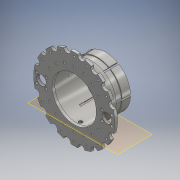
# Autodesk Inventor part: Fixture
Saved by Autodesk Inventor 2016 (Build 200138000, 138)
## iProperties
Created: 2015-07-19
Part Number: Fixture
Material: Generic
Document SubType Name: Modeling
Designer: bastli
Density: 1 g/cm^3
Appearance: Aluminum - Polished
Author: bastli
Autodesk Inventor part; units mm, degrees
ref_plane "YZ Plane" through (0, 0, 0) normal (1, 0, 0) x (0, 1, 0)
ref_plane "XZ Plane" through (0, 0, 0) normal (0, 1, 0) x (-1, 0, 0)
sketch "Sketch1" plane through (0, 0, 0) normal (0, 1, 0) x (-1, 0, 0)
  circle A0 centre (0, 0) radius 67.57
  circle A1 centre (0, 0) radius 38.25
  circle A2 centre (0, 0) radius 41.25
  circle A3 centre (0, 0) radius 36.85
  line L0 (67.57, 0) -> (-67.57, 0) construction
  line L1 (0, 67.57) -> (0, -67.57) construction
  line L2 (62.41, -8) -> (46.41, -8) construction
  line L3 (46.41, -8) -> (46.41, 8) construction
  line L4 (46.41, 8) -> (62.41, 8) construction
  line L5 (62.41, 8) -> (62.41, -8) construction
  line L6 (62.41, -8) -> (46.41, 8) construction
  line L7 (46.41, -8) -> (62.41, 8) construction
  line L8 (64.57, -10.16) -> (44.25, -10.16) construction
  line L9 (44.25, -10.16) -> (44.25, 10.16) construction
  line L10 (44.25, 10.16) -> (64.57, 10.16) construction
  line L11 (64.57, 10.16) -> (64.57, -10.16) construction
  line L12 (64.57, -10.16) -> (44.25, 10.16) construction
  line L13 (44.25, -10.16) -> (64.57, 10.16) construction
  line L14 (64.57, 0) -> (67.57, 0) construction
  line L15 (44.25, 0) -> (41.25, 0) construction
  circle A4 centre (54.41, 0) radius 7.995
  circle A5 centre (-54.41, 0) radius 7.995
  point P0 (-62.41, 8)
  point P1 (-46.41, 8)
  point P2 (-46.41, -8)
  point P3 (-62.41, -8)
  dimension "d0" = 135.14
  dimension "d1" = 76.5
  dimension "d2" = 3
  dimension "d3" = 73.7
  dimension "d4" = 16
  dimension "d5" = 16
  dimension "d6" = 20.32
  dimension "d7" = 20.32
  dimension "d30" = 15.99
  constraints: 32 end point, 9 midpoint, 8 coincident, 5 centre point, 5 symmetric about line, 4 parallel, 4 point on circle, 3 horizontal, 2 collinear, 2 perpendicular, 2 point on line, 1 horizontal alignment, 1 vertical, 3 other
  measures "d0" diameter of A0
  measures "d1" diameter of A1
  measures "d3" diameter of A3
  measures "d4" distance of L3.end L4.end
  measures "d5" distance of L4.end L2.start
  measures "d6" distance of L9.end L10.end
  measures "d7" distance of L10.end L8.start
  measures "d30" diameter of A4
extrude "Extrusion1" add sketch "Sketch1" against normal blind 4.5 contours A0 | A1 | A2 | A4 | A5
extrude "Extrusion2" add sketch "Sketch1" along normal blind 48 contours A2
ref_plane "Work Plane1" through (0, 24, 0) normal (0, 1, 0) x (1, 0, 0)
sketch "Sketch2" plane through (0, 24, 0) normal (0, 1, 0) x (1, 0, 0)
  circle A0 centre (0, 0) radius 38.25 projected
  circle A1 centre (0, 0) radius 41.25 projected
  circle A2 centre (0, 0) radius 39.75
  dimension "d14" = 1.5
  constraints: 1 centre point
  measures "d14" radial gap between concentric circles of A1 A2
extrude "Extrusion3" cut sketch "Sketch2" along normal blind 10 contours A1
sketch "Sketch3" plane through (0, 48, 0) normal (0, 1, 0) x (1, 0, 0)
  circle A0 centre (0, 0) radius 41.25 projected
  circle A1 centre (0, 0) radius 38.25 projected
  line L0 (0, 0) -> (41.25, 0) construction
  line L1 (0, 0) -> (41.2249, 1.4396) construction
  circle A2 centre (0, 0) radius 41.25 projected
  line L2 (0, 0) -> (41.2249, -1.4396) construction
  line L3 (41.2249, 1.4396) -> (38.2267, 1.3349)
  circle A3 centre (0, 0) radius 38.25 projected
  line L4 (41.2249, -1.4396) -> (38.2267, -1.3349)
  dimension "d17" = 4
  constraints: 10 end point, 7 point on circle, 2 point on line, 1 horizontal, 1 other
  measures "d17" angle of L2 L1
extrude "Extrusion4" cut sketch "Sketch3" against normal up to surface (24 mm away) contours A0 L4 A1 L3 picked at (40.2301, -1.2448)
pattern_circular "Circular Pattern1" count 6 over 360 about axis through (0, 0, 0) along (0, 1, 0) of "Extrusion4"
fillet "Fillet1" radius 3 1 edges at (41.25, 0, 0)
hole "Hole1" at (-62.41, 0, 8) at (-46.41, 0, 8) at (-46.41, 0, -8) at (-62.41, 0, -8) at (62.41, 0, 8) at (46.41, 0, 8) at (46.41, 0, -8) at (62.41, 0, -8) direction (0, -1, 0) diameter 2.4 end through all
extrude "Extrusion5" cut sketch "Sketch1" against normal through all contours A4 | A5
sketch "Sketch4" plane through (0, -4.5, 0) normal (0, -1, 0) x (1, 0, 0)
  circle A0 centre (-46.41, -8) radius 1.2 construction
  circle A1 centre (-62.41, 8) radius 1.2 construction
  circle A2 centre (-46.41, 8) radius 1.2 construction
  circle A3 centre (46.41, 8) radius 1.2 construction
  circle A4 centre (46.41, -8) radius 1.2 construction
  circle A5 centre (62.41, -8) radius 1.2 construction
  circle A6 centre (62.41, 8) radius 1.2 construction
  circle A7 centre (-62.41, -8) radius 1.2 construction
  point P0 (0, 0)
  constraints: 8 coincident
hole "Hole2" at (-62.41, -4.5, 8) at (-46.41, -4.5, 8) at (-46.41, -4.5, -8) at (-62.41, -4.5, -8) at (46.41, -4.5, -8) at (46.41, -4.5, 8) at (62.41, -4.5, 8) at (62.41, -4.5, -8) direction (0, 1, 0) diameter 4.4 depth 3 tip angle 118
sketch "Sketch5" plane through (0, 0, 0) normal (0, 1, 0) x (1, 0, 0)
  circle A0 centre (-54.41, 0) radius 7.995 construction
  circle A1 centre (54.41, 0) radius 7.995 construction
  circle A2 centre (46.41, 8) radius 1.2 construction
  circle A3 centre (62.41, -8) radius 1.2 construction
  circle A4 centre (-46.41, 8) radius 1.2 construction
  circle A5 centre (-62.41, -8) radius 1.2 construction
  circle A6 centre (-46.41, -8) radius 1.2 construction
  circle A7 centre (-62.41, 8) radius 1.2 construction
  circle A8 centre (46.41, -8) radius 1.2 construction
  circle A9 centre (62.41, 8) radius 1.2 construction
  circle A10 centre (0, 0) radius 67.57 construction
  circle A11 centre (0, 0) radius 44.25 construction
  circle A12 centre (0, 0) radius 61.57 construction
  circle A13 centre (0, 0) radius 47.25 construction
  line L0 (0, -47.25) -> (0, -61.57) construction
  line L1 (0, -47.25) -> (0, 0) construction
  circle A14 centre (54.41, 0) radius 7.995 projected
  circle A15 centre (0, 0) radius 44.25 projected
  line L2 (54.41, 0) -> (0, 0) construction
  point P0 (21.0582, -57.8569)
  point P1 (16.1605, -44.4005)
  point P2 (39.5764, -47.1654)
  point P3 (30.3717, -36.1956)
  point P4 (53.3212, -30.785)
  point P5 (40.9197, -23.625)
  point P6 (-16.1605, -44.4005)
  point P7 (-21.0582, -57.8569)
  point P8 (-30.3717, -36.1956)
  point P9 (-39.5764, -47.1654)
  point P10 (-40.9197, -23.625)
  point P11 (-53.3212, -30.785)
  point P12 (0, 61.57)
  point P13 (0, 47.25)
  point P14 (21.0582, 57.8569)
  point P15 (16.1605, 44.4005)
  point P16 (39.5764, 47.1654)
  point P17 (30.3717, 36.1956)
  point P18 (53.3212, 30.785)
  point P19 (40.9197, 23.625)
  point P20 (-16.1605, 44.4005)
  point P21 (-21.0582, 57.8569)
  point P22 (-30.3717, 36.1956)
  point P23 (-39.5764, 47.1654)
  point P24 (-40.9197, 23.625)
  point P25 (-53.3212, 30.785)
  dimension "d40" = 6
  dimension "d41" = 3
  dimension "d44" = 60
  dimension "d48" = 60
  constraints: 14 symmetric about line, 6 end point, 2 vertical, 2 vertical alignment, 1 horizontal, 18 other
hole "Hole3" at (0, 0, 61.57) at (0, 0, 47.25) at (21.0582, 0, 57.8569) at (16.1605, 0, 44.4005) at (39.5764, 0, 47.1654) at (30.3717, 0, 36.1956) at (53.3212, 0, 30.785) at (40.9197, 0, 23.625) at (-16.1605, 0, 44.4005) at (-21.0582, 0, 57.8569) at (-30.3717, 0, 36.1956) at (-39.5764, 0, 47.1654) at (-40.9197, 0, 23.625) at (-53.3212, 0, 30.785) at (40.9197, 0, -23.625) at (53.3212, 0, -30.785) at (39.5764, 0, -47.1654) at (30.3717, 0, -36.1956) at (16.1605, 0, -44.4005) at (21.0582, 0, -57.8569) at (0, 0, -47.25) at (0, 0, -61.57) at (-21.0582, 0, -57.8569) at (-16.1605, 0, -44.4005) at (-30.3717, 0, -36.1956) at (-39.5764, 0, -47.1654) at (-40.9197, 0, -23.625) at (-53.3212, 0, -30.785) direction (0, -1, 0) diameter 3.1 end through all
ref_plane "Work Plane2" through (0, 0, -41.25) normal (0, 0, 1) x (1, 0, 0)
sketch "Sketch6" plane through (0, 0, -41.25) normal (0, 0, 1) x (1, 0, 0)
  line L0 (0, 0) -> (0, 6) construction
  dimension "d57" = 6
  constraints: 2 end point, 1 vertical
  measures "d57" distance of L0.start L0.end
hole "Hole4" at (0, 6, -41.25) direction (0, 0, 1) diameter 6 end through all
sketch "Sketch7" plane through (0, 0, 0) normal (0, 1, 0) x (1, 0, 0)
  circle A0 centre (0, 0) radius 67.57 projected
  circle A1 centre (11.7334, -66.5435) radius 6
  line L0 (0, 0) -> (0, -67.57) construction
  line L1 (11.7334, -66.5435) -> (0, 0) construction
  dimension "d65" = 12
  dimension "d66" = 10
  constraints: 4 end point, 2 point on circle, 1 centre point, 1 vertical
  measures "d65" diameter of A1
  measures "d66" angle of L0 L1
extrude "Extrusion6" cut sketch "Sketch7" against normal up to surface (4.5 mm away) contours A1 A0 | A0 A1 picked at (11.6158, -64.5273) picked at (12.0898, -68.4914)
pattern_circular "Circular Pattern2" count 4 over 60 about axis through (0, 0, 0) along (0, 1, 0) of "Extrusion6"
mirror "Mirror2" about plane through (0, 0, 0) normal (1, 0, 0) of "Extrusion6", "Circular Pattern2"
mirror "Mirror3" about plane through (0, 0, 0) normal (0, 0, 1) of "Extrusion6", "Circular Pattern2", "Mirror2"
equation "\"d0\" = outer_radius"
equation "\"d1\" = pvc_radius"
equation "\"d2\" = thickness"
equation "\"d3\" = pcv_foot_radius"
equation "\"d4\" = nema_8_hole_distance"
equation "\"d5\" = nema_8_hole_distance"
equation "\"d6\" = nema_8_width"
equation "\"d7\" = nema_8_width"
equation "\"d8\" = 1.5 * thickness"
equation "\"d10\" = fixture_height"
equation "\"d14\" = 0.5 * thickness"
equation "\"d38\" = thickness"
equation "\"d40\" = 2 * thickness"
equation "\"d41\" = thickness"
equation "\"d57\" = 2 * thickness"
equation "\"thickness\" = 3"
equation "\"outer_radius\" = 6 * thickness + pvc_radius + 2 * nema_8_width"
equation "\"pvc_radius\" = 76.5"
equation "\"pcv_foot_radius\" = 73.7"
equation "\"nema_8_width\" = 20.32"
equation "\"nema_8_hole_distance\" = 16"
equation "\"fixture_height\" = 16 * thickness"
equation "\"d13\" = 0.5 * fixture_height"
equation "\"m3_through\" = 3.4"
equation "\"m3_head\" = 6"
equation "\"m3_hold\" = 3.1"
body "Solid1"
